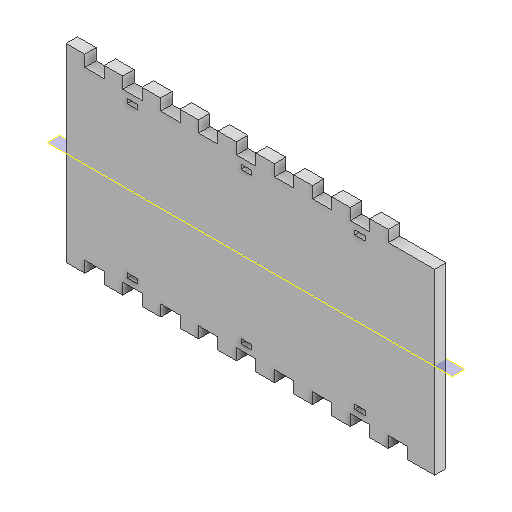
# Autodesk Inventor part: 00_Baseplate_Simmo_side5_v2
Saved by Autodesk Inventor 2024.1 (Build 281209000, 209)
## iProperties
Created: 2022-08-09
Part Number: 00_Baseplate_Simmo_side5_v2
Material: Generic
Document SubType Name: Modeling
Designer: wanghaoran
Density: 1 g/cm^3
Appearance: Default
Author: wanghaoran
Autodesk Inventor part; units mm, degrees
ref_plane "YZ Plane" through (0, 0, 0) normal (1, 0, 0) x (0, 1, 0)
ref_plane "XZ Plane" through (0, 0, 0) normal (0, 1, 0) x (-1, 0, 0)
ref_plane "XY Plane" through (0, 0, 0) normal (0, 0, 1) x (1, 0, 0)
sketch "Sketch1" plane through (0, 0, 0) normal (0, 0, 1) x (1, 0, 0)
  line L0 (184.3024, 11) -> (184.3024, 17) projected
  line L1 (-10, 11) -> (-10, 17) projected
  line L2 (184.3024, 17) -> (0, 17)
  line L3 (0, 17) -> (0, -83)
  line L4 (0, -83) -> (184.3024, -83)
  line L5 (184.3024, -83) -> (184.3024, 17)
  line L6 (-10, 17) -> (0, 17)
  line L7 (0, 17) -> (0, -83)
  line L8 (0, -83) -> (-10, -83)
  line L9 (-10, -83) -> (-10, 17)
  point P0 (0, 0)
  point P1 (-10, 6)
  point P2 (-10, 0)
  dimension "d0" = 100
  constraints: 16 end point, 4 parallel, 2 horizontal, 2 perpendicular
  measures "d0" distance of L3.end L2.end
extrude "Extrusion1" add sketch "Sketch1" along normal blind 6
sketch "Sketch4" plane through (0, 0, 6) normal (0, 0, 1) x (1, 0, 0)
  line L0 (160, 11) -> (184.3024, 11) projected
  line L1 (160, 17) -> (160, 11) projected
  line L2 (184.3024, 17) -> (-10, 17) projected
  line L3 (184.3024, -83) -> (184.3024, 17) projected
  line L4 (0, 11) -> (-10, 11) projected
  line L5 (0, 17) -> (0, 0) projected
  line L6 (-10, 17) -> (-10, -83) projected
  point P0 (-10, 11)
extrude "Extrusion4" cut sketch "Sketch4" against normal blind 6 contours L1 L2 L3 L0
sketch "Sketch5" plane through (0, 0, 6) normal (0, 0, 1) x (1, 0, 0)
  line L0 (140, 11) -> (150, 11) projected
  line L1 (150, 11) -> (150, 17) projected
  line L2 (140, 17) -> (140, 11) projected
  line L3 (184.3024, 17) -> (-10, 17) projected
  line L4 (150, 11) -> (150.1, 11)
  line L5 (150.1, 11) -> (150.1, 17)
  line L6 (150.1, 17) -> (150, 17)
  line L7 (150, 17) -> (150, 11)
  line L8 (140, 11) -> (139.9, 11)
  line L9 (139.9, 11) -> (139.9, 17)
  line L10 (139.9, 17) -> (140, 17)
  line L11 (140, 17) -> (140, 11)
  point P0 (0, 0)
  point P1 (160, 17)
  point P2 (0, 6)
  point P3 (150.1, 17)
  point P4 (139.9, 17)
  point P5 (-10, 17)
  point P6 (184.3024, 17)
  dimension "d21" = 0.1
  dimension "d22" = 6
  dimension "d23" = 0.1
  dimension "d24" = 6
  constraints: 16 end point, 4 parallel, 2 horizontal, 2 perpendicular, 1 other
  measures "d21" distance of L6.end L5.end
  measures "d22" distance of L5.end L4.end
  measures "d23" distance of L9.end L10.end
  measures "d24" distance of L8.end L9.end
extrude "Extrusion5" cut sketch "Sketch5" against normal blind 6
pattern_linear "Rectangular Pattern3" count 8 spacing 20 along (-1, 0, 0) of "Extrusion5"
ref_plane "Work Plane1" through (-10, -33, 0) normal (0, -1, 0) x (1, 0, 0)
mirror "Mirror1" about plane through (-10, -33, 0) normal (0, -1, 0) of "Extrusion5"
pattern_linear "Rectangular Pattern4" count 2 spacing 20 along (1, 0, 0) count 8 spacing 20 along (-1, 0, 0) of "Extrusion5", "Mirror1"
sketch "Sketch6" plane through (0, 0, 6) normal (0, 0, 1) x (1, 0, 0)
  line L0 (167.75, 6.6) -> (162.25, 6.6)
  line L1 (162.25, 6.6) -> (162.25, 9)
  line L2 (162.25, 9) -> (167.75, 9)
  line L3 (167.75, 9) -> (167.75, 6.6)
  line L4 (159.9, 11) -> (159.9, 17) projected
  line L5 (184.3024, 11) -> (160, 11) projected
  line L6 (147.75, 5.6) -> (142.25, 5.6)
  line L7 (142.25, 5.6) -> (142.25, 8)
  line L8 (142.25, 8) -> (147.75, 8)
  line L9 (147.75, 8) -> (147.75, 5.6)
  line L10 (150.1, 11) -> (139.9, 11) projected
  line L11 (139.9, 11) -> (139.9, 17) projected
  point P0 (0, 0)
  dimension "d36" = 5.5
  dimension "d37" = 2.4
  dimension "d38" = 2.35
  dimension "d39" = 2
  dimension "d48" = 5.5
  dimension "d49" = 2.4
  dimension "d50" = 3
  dimension "d51" = 2.35
  constraints: 16 end point, 4 parallel, 2 horizontal, 2 perpendicular
  measures "d36" distance of L1.end L2.end
  measures "d37" distance of L0.end L1.end
  measures "d38" distance between parallel lines of L4 L1
  measures "d39" distance between parallel lines of L5 L2
  measures "d48" distance of L7.end L8.end
  measures "d49" distance of L6.end L7.end
  measures "d50" distance between parallel lines of L10 L8
  measures "d51" distance between parallel lines of L11 L7
extrude "Extrusion6" cut sketch "Sketch6" against normal blind 6 contours L6 L7 L8 L9
pattern_linear "Rectangular Pattern5" count 3 spacing 60 along (-1, 0, 0) of "Extrusion6"
mirror "Mirror2" about plane through (-10, -33, 0) normal (0, -1, 0) of "Extrusion6", "Rectangular Pattern5"
body "Solid1"
